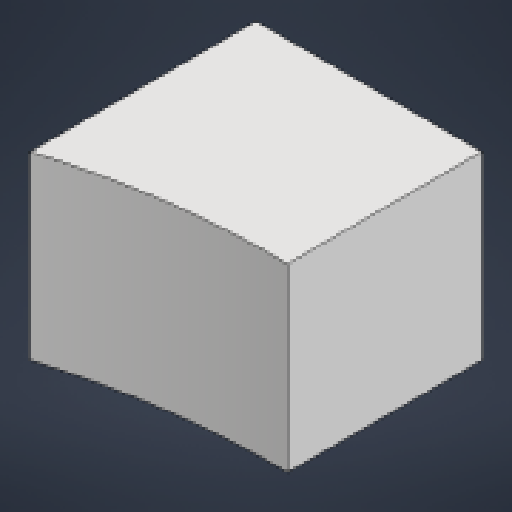
# Autodesk Inventor part: 3DPRINT,BLOCK,LEFT
Saved by Autodesk Inventor 2026.1 (Build 301233020, 233B)
## iProperties
Created: 2026-03-19
Part Number: 3DPRINT,BLOCK,LEFT
Material: Generic
Document SubType Name: Modeling
Designer: Owen L
Density: 1 g/cm^3
Appearance: Default
Author: Owen L
Autodesk Inventor part; units mm, degrees
ref_plane "YZ Plane" through (0, 0, 0) normal (1, 0, 0) x (0, 1, 0)
ref_plane "XZ Plane" through (0, 0, 0) normal (0, 1, 0) x (-1, 0, 0)
ref_plane "XY Plane" through (0, 0, 0) normal (0, 0, 1) x (1, 0, 0)
sketch "Sketch1" plane through (0, 0, 0) normal (0, 0, 1) x (1, 0, 0)
  line L0 (-63.5, 50.8) -> (63.5, 50.8)
  line L1 (63.5, 50.8) -> (63.5, -50.8)
  line L2 (63.5, -50.8) -> (-63.5, -50.8)
  line L3 (-63.5, -50.8) -> (-63.5, 50.8)
  line L4 (-63.5, 50.8) -> (63.5, -50.8) construction
  line L5 (63.5, 50.8) -> (-63.5, -50.8) construction
  point P0 (0, 0)
  dimension "d0" = 101.6
  dimension "d1" = 127
  constraints: 12 end point, 2 midpoint, 2 parallel, 1 horizontal, 1 perpendicular
  measures "d0" distance of L2.end L0.start
  measures "d1" distance of L1.end L2.end
extrude "Extrusion1" add sketch "Sketch1" along normal blind 127
sketch "Sketch2" plane through (-63.5, 50.8, 0) normal (0, 1, 0) x (1, 0, 0)
  arc A0 (127, -109.22) -> (0, -127) centre (119.1408, -515.544) ccw
  line L0 (127, -127) -> (0, -127) projected
  line L1 (127, 0) -> (127, -127) projected
  line L2 (127, -109.22) -> (127, -127)
  line L3 (127, -127) -> (0, -127)
  point P0 (63.5, 0)
  dimension "d4" = 406.4
  dimension "d5" = 17.78
  constraints: 4 end point, 3 point on circle, 2 collinear, 1 centre point, 1 point on line
  measures "d4" radius of A0
  measures "d5" distance from line of L0 L2.start
extrude "Extrusion2" cut sketch "Sketch2" against normal through all
body "Solid1"
